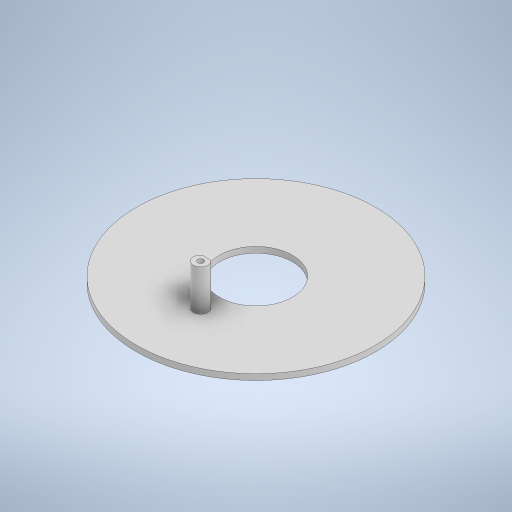
# Autodesk Inventor part: lidbetter
Saved by Autodesk Inventor 2024 (Build 280153000, 153)
## iProperties
Created: 2024-05-20
Part Number: lidbetter
Material: Generic
Document SubType Name: Modeling
Designer: ryana
Density: 1 g/cm^3
Appearance: Default
Author: ryana
Autodesk Inventor part; units mm, degrees
ref_plane "YZ Plane" through (0, 0, 0) normal (1, 0, 0) x (0, 1, 0)
ref_plane "XZ Plane" through (0, 0, 0) normal (0, 1, 0) x (-1, 0, 0)
ref_plane "XY Plane" through (0, 0, 0) normal (0, 0, 1) x (1, 0, 0)
sketch "Sketch1" plane through (0, 0, 0) normal (0, 1, 0) x (-1, 0, 0)
  circle A0 centre (0, 0) radius 41
  circle A1 centre (0, 0) radius 12.5
  dimension "d0" = 82
  dimension "d1" = 25
  constraints: 2 centre point, 2 coincident
  measures "d0" diameter of A0
  measures "d1" diameter of A1
extrude "Extrusion1" add sketch "Sketch1" along normal blind 2
sketch "Sketch2" plane through (0, 2, 0) normal (0, 1, 0) x (1, 0, 0)
  line L0 (0, 0) -> (0, -19)
  line L1 (0, 0) -> (19, 0) construction
  circle A0 centre (0, -19) radius 2.5
  dimension "d4" = 19
  dimension "d5" = 90
  dimension "d6" = 5
  constraints: 4 end point, 1 centre point, 1 coincident, 1 horizontal, 1 perpendicular, 1 vertical
  measures "d4" distance of L0.start L0.end
  measures "d5" angle of L0 L1
  measures "d6" diameter of A0
extrude "Extrusion2" add sketch "Sketch2" along normal blind 14
sketch "Sketch3" plane through (0, 16, 19) normal (0, 1, 0) x (1, 0, 0)
  circle A0 centre (0, 0) radius 2.5 projected
  circle A1 centre (0, 0) radius 1
  point P0 (0, 19)
  dimension "d9" = 2
  constraints: 1 centre point, 1 coincident
  measures "d9" diameter of A1
extrude "Extrusion3" cut sketch "Sketch3" against normal blind 14 contours A1
sketch "Sketch4" plane through (0, 16, 19) normal (0, 1, 0) x (1, 0, 0)
  circle A0 centre (0, 0) radius 1 projected
  line L0 (0, 0) -> (0, 2.5)
  circle A1 centre (0, 0) radius 2.5 projected
  line L1 (0, 2.5) -> (0, 2)
  line L2 (0, 2) -> (-3, 2)
  line L3 (-3, 2) -> (-3, 2.5)
  line L4 (-3, 2.5) -> (0, 2.5)
  line L5 (0, 2.5) -> (0, 2)
  line L6 (0, 2) -> (3, 2)
  line L7 (3, 2) -> (3, 2.5)
  line L8 (3, 2.5) -> (0, 2.5)
  point P0 (0, 19)
  point P1 (-1.5, 2)
  dimension "d12" = 0.5
  dimension "d13" = 3
  dimension "d14" = 0.5
  dimension "d15" = 3
  constraints: 18 end point, 4 parallel, 2 perpendicular, 2 point on circle, 1 collinear, 1 point on line, 1 vertical
  measures "d12" distance of L0.end L1.end
  measures "d13" distance of L1.end L2.end
  measures "d14" distance of L5.start L1.end
  measures "d15" distance of L6.end L1.end
extrude "Extrusion4" cut sketch "Sketch4" against normal blind 14 contours L2 A1 L0 | L0 A1 L6 | L8 L7 L6 A1
body "Solid1"
